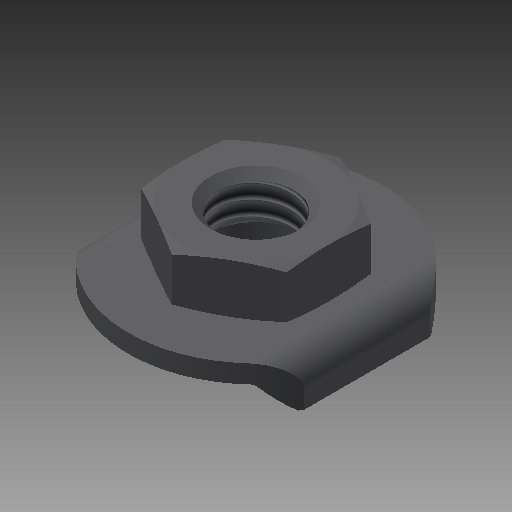
# Autodesk Inventor part: 102111-M-KOMP
Saved by Autodesk Inventor 2018 (Build 220112000, 112)
## iProperties
Category: PARTsolutions
Company: DESTACO
Created: 2018-01-28
Part Number: 102111-M-KOMP
Catalog Web Link: www.cadenas.de
Description: 102111-M-KOMP-Flankenscheibe
Vendor: DESTACO
Document SubType Name: Modeling
Designer: psAdmin
Manufacturer: DESTACO
Mass: 0.241963 g
Surface Area: 4.6208 cm^2
Volume: 0.241963 cm^3
Density: 1 g/cm^3
Material: Generic
Appearance: PSOLRGB-192-192-192
PSOL_IDENT_0: {$CADENAS_DATA\23d-libs\destaco\destaco_gmbh\man_spann\horizontalspanner\kompakt\u_kompakt_parts\fla
PSOL_IDENT_1: nkenscheibe_u_komp.prj},168 {VTYP=3D},{NB=102111-M-KOMP},{LINA=102111-M-KOMP},{NN=102111-M-KOMP},{DA
PSOL_IDENT_2: TE=20.09.2016 07:53:11},{GEOMDATE=16.03.2006},{VERSION=v1},{LINEID=10},{LINESUBID=-1},{WBVAR=}  {NB=
PSOL_IDENT_3: 102111-M-KOMP},{LINA=102111-M-KOMP},{KT=DUMMY},{MODELL=102111-M-KOMP},{SIZE=1.000},{VER=1}
NN: 102111-M-KOMP
NT: Flankenscheibe
NB: 102111-M-KOMP
NBSYN: $MODELL.
LINA: 102111-M-KOMP
MODELL: 102111-M-KOMP
SUPPLIER: DESTACO
ARTICLENO: 102111-M-KOMP
BOMINFO: 102111-M-KOMP
CREATOR: CADENAS GmbH
Title: 102111-M-KOMP
Author: Cadenas PARTsolutions
Comments: Flankenscheibe
Autodesk Inventor part; units mm, degrees
sketch "Skizze_1" plane through (0, 0, 0) normal (0, 0, 1) x (1, 0, 0)
  line L0 (-6.094, 2.6187) -> (-5.9701, 2.6187)
  line L1 (-5.9701, 2.6187) -> (-4.9601, 3.9225)
  arc A0 (-4.8019, 4) -> (-4.9601, 3.9225) centre (-4.8019, 3.8) ccw
  line L2 (-4.8019, 4) -> (4.8019, 4)
  arc A1 (4.9601, 3.9225) -> (4.8019, 4) centre (4.8019, 3.8) ccw
  line L3 (4.9601, 3.9225) -> (5.9701, 2.6187)
  line L4 (5.9701, 2.6187) -> (6.094, 2.6187)
  line L5 (6.094, 2.6187) -> (6.094, 3.606)
  arc A2 (6.094, 3.606) -> (4.7, 5) centre (4.7, 3.606) ccw
  line L6 (4.7, 5) -> (-4.7, 5)
  arc A3 (-4.7, 5) -> (-6.094, 3.606) centre (-4.7, 3.606) ccw
  line L7 (-6.094, 3.606) -> (-6.094, 2.6187)
  constraints: 16 end point, 8 point on circle, 4 centre point
extrude "Extrusion1" add sketch "Skizze_1" along normal mid plane 14
sketch "Skizze_2" plane through (0, 0, 0) normal (0, 0, 1) x (1, 0, 0)
  line L0 (0, 5) -> (0, 7.7)
  line L1 (0, 7.7) -> (4, 7.7)
  line L2 (4, 7.7) -> (4.8, 7.4856)
  line L3 (4.8, 7.4856) -> (4.8, 5.2144)
  line L4 (4.8, 5.2144) -> (4, 5)
  line L5 (4, 5) -> (0, 5)
  line L6 (0, 5) -> (0, 7.7)
  constraints: 14 end point
revolve "Revolution1" add sketch "Skizze_2" angle 360 about axis through (0, 5, 0) along (0, -1, 0)
sketch "Skizze_3" plane through (0, 5, 0) normal (0, 1, 0) x (1, 0, 0)
  line L0 (-20, -18) -> (19, -18)
  line L1 (19, -18) -> (19, 12)
  line L2 (19, 12) -> (-20, 12)
  line L3 (-20, 12) -> (-20, -18)
  line L4 (-4, -2.3094) -> (0, -4.6188)
  line L5 (0, -4.6188) -> (4, -2.3094)
  line L6 (4, -2.3094) -> (4, 2.3094)
  line L7 (4, 2.3094) -> (0, 4.6188)
  line L8 (0, 4.6188) -> (-4, 2.3094)
  line L9 (-4, 2.3094) -> (-4, -2.3094)
  constraints: 20 end point
extrude "Extrusion2" cut sketch "Skizze_3" along normal blind 2.7
sketch "Skizze_4" plane through (0, 0, 0) normal (0, 1, 0) x (-1, 0, 0)
  line L0 (23, 26) -> (-35, 26)
  line L1 (-35, 26) -> (-35, -16)
  line L2 (-35, -16) -> (23, -16)
  line L3 (23, -16) -> (23, 26)
  circle A0 centre (0, 0) radius 7
  constraints: 8 end point, 1 centre point
extrude "Extrusion3" cut sketch "Skizze_4" along normal blind 10
sketch "Skizze_5_ALT_Drilling_1" plane through (0, 0, 0) normal (0, 0, 1) x (1, 0, 0)
  line L0 (0, 4) -> (0, 7.7)
  line L1 (0, 7.7) -> (2.5, 7.7)
  line L2 (2.5, 7.7) -> (2.067, 7.267)
  line L3 (2.067, 7.267) -> (2.067, 5.433)
  line L4 (2.067, 5.433) -> (2.5, 5)
  line L5 (2.5, 5) -> (2.65, 5)
  line L6 (2.65, 5) -> (2.65, 4)
  line L7 (2.65, 4) -> (0, 4)
  line L8 (0, 4) -> (0, 7.7)
  constraints: 18 end point
revolve "Revolution2" cut sketch "Skizze_5_ALT_Drilling_1" angle 360 about axis through (0, 4, 0) along (0, -1, 0)
thread "Thread1" size "M5x0.8" class "6H" standard "ISO Metric profile" full length
ref_plane "FS1_XY" through (0, 0, 0) normal (0, 1, 0) x (1, 0, 0)
ref_plane "FS1_YZ" through (0, 0, 0) normal (1, 0, 0) x (0, 0, -1)
ref_plane "FS1_ZX" through (0, 0, 0) normal (0, 0, -1) x (0, 1, 0)
ref_plane "FS2_XY" through (0, 0, 0) normal (0, 0, 1) x (1, 0, 0)
ref_plane "FS2_YZ" through (0, 0, 0) normal (1, 0, 0) x (0, 1, 0)
ref_plane "FS2_ZX" through (0, 0, 0) normal (0, 1, 0) x (0, 0, 1)
body "Solid1"
